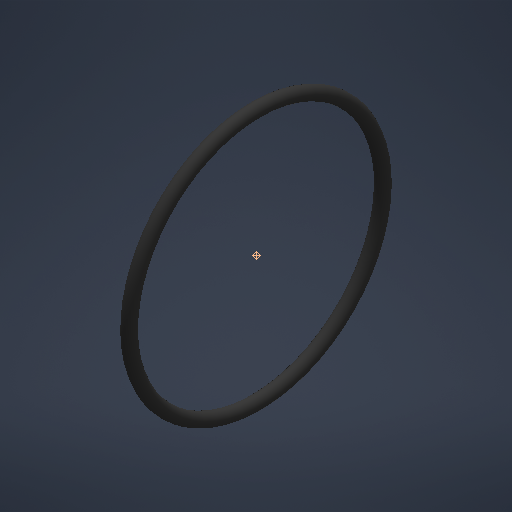
# Autodesk Inventor part: Rodinha-Borracha
Saved by Autodesk Inventor 2026 (Build 300175000, 175)
## iProperties
Created: 2018-07-04
Part Number: Rodinha-Borracha
Material: Borracha
Document SubType Name: Modeling
Designer: Marcelo
Density: 0.93 g/cm^3
Appearance: Borracha - Preta
Author: Marcelo
Autodesk Inventor part; units mm, degrees
ref_plane "YZ Plane" through (0, 0, 0) normal (1, 0, 0) x (0, 1, 0)
ref_plane "XZ Plane" through (0, 0, 0) normal (0, 1, 0) x (-1, 0, 0)
ref_plane "XY Plane" through (0, 0, 0) normal (0, 0, 1) x (1, 0, 0)
sketch "Esboço1" plane through (0, 0, 0) normal (0, 0, 1) x (1, 0, 0)
  line L0 (0, 0) -> (-5.0552, 0)
  line L1 (0, 0) -> (0, 60)
  circle A0 centre (0, 60) radius 3
  dimension "d0" = 60
  dimension "d1" = 6
  constraints: 4 end point, 1 centre point, 1 coincident, 1 horizontal, 1 vertical
  measures "d0" distance of L0.start L1.end
  measures "d1" diameter of A0
revolve "Revolução1" add sketch "Esboço1" angle 360 about axis through (0, 0, 0) along (-1, 0, 0)
